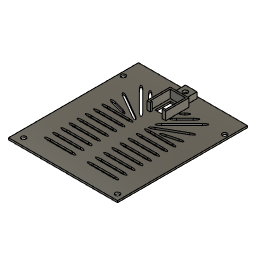
CaseBack (Autodesk Fusion 360 design; units mm, degrees)
Autodesk Fusion 360 part; units mm, degrees
(part 1 of 4)
sketch "Sketch1" plane through (0, 0, 0) normal (0, 0, 1) x (1, 0, 0)
  line L0 (0, 0) -> (94, 0)
  line L1 (94, 0) -> (94, 112.05)
  line L2 (94, 112.05) -> (0, 112.05)
  line L3 (0, 112.05) -> (0, 0)
  line L4 (0, 112.05) -> (3.5, 112.05)
  line L5 (3.5, 112.05) -> (3.5, 95.55)
  line L6 (3.5, 95.55) -> (0, 95.55)
  line L7 (0, 95.55) -> (0, 112.05)
  circle A0 centre (3.5, 95.55) radius 2
  line L8 (94, 112.05) -> (90.5, 112.05)
  line L9 (90.5, 112.05) -> (90.5, 95.55)
  line L10 (90.5, 95.55) -> (94, 95.55)
  line L11 (94, 95.55) -> (94, 112.05)
  circle A1 centre (90.5, 95.55) radius 2
  line L12 (0, 0) -> (5, 0)
  line L13 (5, 0) -> (5, 5)
  line L14 (5, 5) -> (0, 5)
  line L15 (0, 5) -> (0, 0)
  circle A2 centre (5, 5) radius 2
  line L16 (94, 0) -> (87.5, 0)
  line L17 (87.5, 0) -> (87.5, 6.5)
  line L18 (87.5, 6.5) -> (94, 6.5)
  line L19 (94, 6.5) -> (94, 0)
  circle A3 centre (87.5, 6.5) radius 2
  line L20 (0, 112.05) -> (0.25, 112.05)
  line L21 (0.25, 112.05) -> (0.25, 111.8)
  line L22 (0.25, 111.8) -> (0, 111.8)
  line L23 (0, 111.8) -> (0, 112.05)
  line L24 (94, 0) -> (93.75, 0)
  line L25 (93.75, 0) -> (93.75, 0.25)
  line L26 (93.75, 0.25) -> (94, 0.25)
  line L27 (94, 0.25) -> (94, 0)
  line L28 (93.75, 0.25) -> (0.25, 0.25)
  line L29 (0.25, 0.25) -> (0.25, 111.8)
  line L30 (0.25, 111.8) -> (93.75, 111.8)
  line L31 (93.75, 111.8) -> (93.75, 0.25)
  dimension "d1" = 94
  dimension "d2" = 112.05
  dimension "d3" = 3.5
  dimension "d4" = 16.5
  dimension "d5" = 4
  dimension "d6" = 3.5
  dimension "d7" = 16.5
  dimension "d8" = 4
  dimension "d9" = 5
  dimension "d10" = 5
  dimension "d11" = 4
  dimension "d12" = 6.5
  dimension "d13" = 6.5
  dimension "d14" = 4
  dimension "d15" = 0.25
  dimension "d16" = 0.25
  dimension "d17" = 0.25
  dimension "d18" = 0.25
  constraint horizontal L0
  constraint vertical L1
  constraint horizontal L2
  constraint vertical L3
  constraint horizontal L4
  constraint vertical L5
  constraint horizontal L6
  constraint vertical L7
  constraint coincident L5.end L6.start
  constraint horizontal L8
  constraint vertical L9
  constraint horizontal L10
  constraint vertical L11
  constraint coincident L9.end L10.start
  constraint horizontal L12
  constraint vertical L13
  constraint horizontal L14
  constraint vertical L15
  constraint coincident L13.end L14.start
  constraint horizontal L16
  constraint vertical L17
  constraint horizontal L18
  constraint vertical L19
  constraint coincident L17.end L18.start
  constraint horizontal L20
  constraint vertical L21
  constraint horizontal L22
  constraint vertical L23
  constraint horizontal L24
  constraint vertical L25
  constraint horizontal L26
  constraint vertical L27
  constraint horizontal L28
  constraint vertical L29
  constraint horizontal L30
  constraint vertical L31
  measures "d1" distance of L0.start L0.end
  measures "d2" distance of L0.start L2.end
  measures "d3" distance of L2.end L4.end
  measures "d4" distance of L2.end L6.end
  measures "d5" diameter of A0
  measures "d6" distance of L1.end L8.end
  measures "d7" distance of L1.end L10.end
  measures "d8" diameter of A1
  measures "d9" distance of L0.start L12.end
  measures "d10" distance of L0.start L14.end
  measures "d11" diameter of A2
  measures "d12" distance of L0.end L16.end
  measures "d13" distance of L0.end L18.end
  measures "d14" diameter of A3
  measures "d15" distance of L2.end L20.end
  measures "d16" distance of L2.end L22.end
  measures "d17" distance of L0.end L24.end
  measures "d18" distance of L0.end L26.end
extrude "Extrude1" add sketch "Sketch1" along normal blind 1.5 contours L13 L14 A2 L28 L29 | L5 L6 A0 L9 L10 A1 L13 L14 A2 L17 L18 A3 L28 L29 L30 L31 | L17 L18 A3 L28 L31 | L5 L6 A0 L29 L30 | L9 L10 A1 L30 L31
sketch "Sketch2" plane through (0, 0, 1.5) normal (0, 0, 1) x (-1, 0, 0)
  circle A0 centre (-87.5, -6.5) radius 2
  circle A1 centre (-90.5, -95.55) radius 2
  circle A2 centre (-3.5, -95.55) radius 2
  circle A3 centre (-5, -5) radius 2
  line L0 (-93.75, -111.8) -> (-0.25, -111.8)
  line L1 (-0.25, -111.8) -> (-0.25, -0.25)
  line L2 (-0.25, -0.25) -> (-93.75, -0.25)
  line L3 (-93.75, -0.25) -> (-93.75, -111.8)
  line L4 (-3.5, -95.55) -> (-8.5, -95.55)
  line L5 (-5, -5) -> (-10, -5)
  line L6 (-10, -5) -> (-10, -95.55)
  line L7 (-10, -95.55) -> (-8.5, -95.55)
  line L8 (-10, -111.8) -> (-10, -106.8)
  line L9 (-87.5, -6.5) -> (-82.5, -6.5)
  line L10 (-90.5, -95.55) -> (-85.5, -95.55)
  line L11 (-82.5, -6.5) -> (-82.5, -95.55)
  line L12 (-82.5, -95.55) -> (-85.5, -95.55)
  line L13 (-82.5, -111.8) -> (-82.5, -106.8)
  line L14 (-10, -106.8) -> (-82.5, -106.8)
  line L15 (-82.5, -106.8) -> (-82.5, -6.5)
  line L16 (-82.5, -6.5) -> (-10, -6.5)
  line L17 (-10, -6.5) -> (-10, -106.8)
  line L18 (-82.5, -6.5) -> (-82.5, -0.25)
  line L19 (-82.5, -0.25) -> (-82.5, -5.25)
  line L20 (-82.5, -5.25) -> (-10, -5.25)
  line L21 (-10, -5.25) -> (-10, -6.5)
  line L22 (-10, -6.5) -> (-82.5, -6.5)
  line L23 (-82.5, -6.5) -> (-82.5, -5.25)
  dimension "d21" = 5
  dimension "d22" = 5
  dimension "d23" = 5
  dimension "d24" = 5
  dimension "d25" = 5
  dimension "d26" = 5
  constraint coincident A2.centre L4.start
  constraint horizontal L4
  constraint coincident A3.centre L5.start
  constraint horizontal L5
  constraint perpendicular L4 L6
  constraint perpendicular L6 L7
  constraint coincident L0 L8.start
  constraint perpendicular L0 L8
  constraint coincident A0.centre L9.start
  constraint horizontal L9
  constraint coincident A1.centre L10.start
  constraint horizontal L10
  constraint perpendicular L10 L11
  constraint perpendicular L11 L12
  constraint coincident L0 L13.start
  constraint perpendicular L0 L13
  constraint horizontal L14
  constraint vertical L15
  constraint horizontal L16
  constraint vertical L17
  constraint coincident L2 L18.end
  constraint perpendicular L2 L18
  constraint perpendicular L2 L19
  constraint horizontal L20
  constraint vertical L21
  constraint horizontal L22
  constraint vertical L23
  measures "d21" distance of A2.centre L4.end
  measures "d22" distance of L8.start L8.end
  measures "d23" distance of A0.centre L9.end
  measures "d24" distance of A1.centre L10.end
  measures "d25" distance of L13.start L13.end
  measures "d26" distance of L18.end L19.end
extrude "Extrude2" cut sketch "Sketch2" against normal blind 12 contours L6 L11 L14 L15 L16 L17 L22 | L6 L16 L18 L20 L21 L22 L23
extrude "Extrude3" add 1 faces at (10, 39.1, 1) along direction (1, 0, 0) blind 72.5
sketch "Sketch3" plane through (0, 0, 1.5) normal (0, 0, 1) x (-1, 0, 0)
  circle A0 centre (-87.5, -6.5) radius 2
  circle A1 centre (-90.5, -95.55) radius 2
  circle A2 centre (-3.5, -95.55) radius 2
  circle A3 centre (-5, -5) radius 2
  line L0 (-93.75, -111.8) -> (-0.25, -111.8)
  line L1 (-0.25, -111.8) -> (-0.25, -0.25)
  line L2 (-0.25, -0.25) -> (-93.75, -0.25)
  line L3 (-93.75, -0.25) -> (-93.75, -111.8)
  line L4 (-0.25, -111.8) -> (-15.25, -111.8)
  line L5 (-15.25, -111.8) -> (-15.25, -0.25)
  line L6 (-15.25, -0.25) -> (-0.25, -0.25)
  line L7 (-0.25, -0.25) -> (-0.25, -111.8)
  line L8 (-93.75, -111.8) -> (-78.75, -111.8)
  line L9 (-78.75, -111.8) -> (-78.75, -0.25)
  line L10 (-78.75, -0.25) -> (-93.75, -0.25)
  line L11 (-93.75, -0.25) -> (-93.75, -111.8)
  line L12 (-78.75, -0.25) -> (-15.25, -0.25)
  line L13 (-15.25, -0.25) -> (-15.25, -15.25)
  line L14 (-15.25, -15.25) -> (-78.75, -15.25)
  line L15 (-78.75, -15.25) -> (-78.75, -0.25)
  line L16 (-15.25, -111.8) -> (-78.75, -111.8)
  line L17 (-78.75, -111.8) -> (-78.75, -96.8)
  line L18 (-78.75, -96.8) -> (-15.25, -96.8)
  line L19 (-15.25, -96.8) -> (-15.25, -111.8)
  line L20 (-47, -96.8) -> (-42.5, -96.8)
  line L21 (-42.5, -96.8) -> (-42.5, -83.8)
  line L22 (-42.5, -83.8) -> (-47, -83.8)
  line L23 (-47, -83.8) -> (-47, -96.8)
  line L24 (-47, -96.8) -> (-51.5, -96.8)
  line L25 (-51.5, -96.8) -> (-51.5, -83.8)
  line L26 (-51.5, -83.8) -> (-47, -83.8)
  line L27 (-47, -83.8) -> (-47, -96.8)
  dimension "d31" = 15
  dimension "d32" = 15
  dimension "d33" = 15
  dimension "d34" = 15
  dimension "d35" = 4.5
  dimension "d36" = 13
  dimension "d37" = 4.5
  dimension "d38" = 13
  constraint horizontal L4
  constraint vertical L5
  constraint horizontal L6
  constraint vertical L7
  constraint coincident L2 L5.end
  constraint coincident L0.end L1.start
  constraint horizontal L8
  constraint vertical L9
  constraint horizontal L10
  constraint vertical L11
  constraint coincident L0.start L3.end
  constraint horizontal L12
  constraint vertical L13
  constraint horizontal L14
  constraint vertical L15
  constraint horizontal L16
  constraint vertical L17
  constraint horizontal L18
  constraint vertical L19
  constraint horizontal L20
  constraint vertical L21
  constraint horizontal L22
  constraint vertical L23
  constraint midpoint L18 L20.start
  constraint horizontal L24
  constraint vertical L25
  constraint horizontal L26
  constraint vertical L27
  measures "d31" distance of L0.end L4.end
  measures "d32" distance of L0.start L8.end
  measures "d33" distance of L9.end L14.end
  measures "d34" distance of L4.end L18.end
  measures "d35" distance of L20.start L20.end
  measures "d36" distance of L20.start L22.end
  measures "d37" distance of L20.start L24.end
  measures "d38" distance of L20.start L22.end
extrude "Extrude4" cut sketch "Sketch3" against normal blind 40 contours L18 L23 L24 L25 L26 L27 | L18 L20 L21 L22 L23 L27
sketch "Sketch4" plane through (0, 0, 1.5) normal (0, 0, 1) x (-1, 0, 0)
  line L0 (-42.5, -83.8) -> (-42.5, -96.8)
  line L1 (-42.5, -96.8) -> (-51.5, -96.8)
  line L2 (-51.5, -96.8) -> (-51.5, -83.8)
  line L3 (-51.5, -83.8) -> (-42.5, -83.8)
  circle A0 centre (-87.5, -6.5) radius 2
  circle A1 centre (-90.5, -95.55) radius 2
  circle A2 centre (-3.5, -95.55) radius 2
  circle A3 centre (-5, -5) radius 2
  line L4 (-93.75, -111.8) -> (-0.25, -111.8)
  line L5 (-0.25, -111.8) -> (-0.25, -0.25)
  line L6 (-0.25, -0.25) -> (-93.75, -0.25)
  line L7 (-93.75, -0.25) -> (-93.75, -111.8)
  line L8 (-42.5, -96.8) -> (-40.5, -96.8)
  line L9 (-40.5, -96.8) -> (-40.5, -98.8)
  line L10 (-40.5, -98.8) -> (-42.5, -98.8)
  line L11 (-42.5, -98.8) -> (-42.5, -96.8)
  line L12 (-51.5, -83.8) -> (-53.5, -83.8)
  line L13 (-53.5, -83.8) -> (-53.5, -81.8)
  line L14 (-53.5, -81.8) -> (-51.5, -81.8)
  line L15 (-51.5, -81.8) -> (-51.5, -83.8)
  line L16 (-40.5, -98.8) -> (-53.5, -98.8)
  line L17 (-53.5, -98.8) -> (-53.5, -81.8)
  line L18 (-53.5, -81.8) -> (-40.5, -81.8)
  line L19 (-40.5, -81.8) -> (-40.5, -98.8)
  line L20 (-40.5, -98.8) -> (-39, -98.8)
  line L21 (-39, -98.8) -> (-39, -100.3)
  line L22 (-39, -100.3) -> (-40.5, -100.3)
  line L23 (-40.5, -100.3) -> (-40.5, -98.8)
  line L24 (-53.5, -81.8) -> (-55, -81.8)
  line L25 (-55, -81.8) -> (-55, -80.3)
  line L26 (-55, -80.3) -> (-53.5, -80.3)
  line L27 (-53.5, -80.3) -> (-53.5, -81.8)
  line L28 (-55, -80.3) -> (-39, -80.3)
  line L29 (-39, -80.3) -> (-39, -100.3)
  line L30 (-39, -100.3) -> (-55, -100.3)
  line L31 (-55, -100.3) -> (-55, -80.3)
  line L32 (-40.5, -81.8) -> (-42, -81.8)
  line L33 (-42, -81.8) -> (-42, -80.3)
  line L34 (-42, -80.3) -> (-40.5, -80.3)
  line L35 (-40.5, -80.3) -> (-40.5, -81.8)
  line L36 (-53.5, -81.8) -> (-52, -81.8)
  line L37 (-52, -81.8) -> (-52, -80.3)
  line L38 (-52, -80.3) -> (-53.5, -80.3)
  line L39 (-53.5, -80.3) -> (-53.5, -81.8)
  dimension "d41" = 2
  dimension "d42" = 2
  dimension "d43" = 2
  dimension "d44" = 2
  dimension "d45" = 1.5
  dimension "d46" = 1.5
  dimension "d47" = 1.5
  dimension "d48" = 1.5
  dimension "d49" = 1.5
  dimension "d50" = 1.5
  constraint horizontal L8
  constraint vertical L9
  constraint horizontal L10
  constraint vertical L11
  constraint coincident L0.end L1.start
  constraint horizontal L12
  constraint vertical L13
  constraint horizontal L14
  constraint vertical L15
  constraint coincident L2.end L3.start
  constraint horizontal L16
  constraint vertical L17
  constraint horizontal L18
  constraint vertical L19
  constraint horizontal L20
  constraint vertical L21
  constraint horizontal L22
  constraint vertical L23
  constraint horizontal L24
  constraint vertical L25
  constraint horizontal L26
  constraint vertical L27
  constraint horizontal L28
  constraint vertical L29
  constraint horizontal L30
  constraint vertical L31
  constraint horizontal L32
  constraint vertical L33
  constraint horizontal L34
  constraint vertical L35
  constraint horizontal L36
  constraint vertical L37
  constraint horizontal L38
  constraint vertical L39
  measures "d41" distance of L0.end L8.end
  measures "d42" distance of L0.end L10.end
  measures "d43" distance of L2.end L12.end
  measures "d44" distance of L2.end L14.end
  measures "d45" distance of L9.end L20.end
  measures "d46" distance of L9.end L22.end
  measures "d47" distance of L13.end L24.end
  measures "d48" distance of L13.end L26.end
  measures "d49" distance of L18.end L32.end
  measures "d50" distance of L13.end L36.end
extrude "Extrude5" add sketch "Sketch4" along normal blind 7 contours L9 L19 L20 L28 L29 L35 | L10 L13 L16 L17 L23 L24 L30 L31 | L20 L21 L22 L23 L29 L30 | L18 L28 L32 L33 L34 L35 | L14 L18 L27 L28 L36 L37 L38 L39 | L24 L25 L26 L27 L28 L31 L39
sketch "Sketch5" plane through (0, 0, 1.5) normal (0, 0, 1) x (-1, 0, 0)
  line L0 (-40.5, -81.8) -> (-42, -81.8)
  line L1 (-42, -81.8) -> (-42, -80.3)
  line L2 (-42, -80.3) -> (-39, -80.3)
  line L3 (-39, -80.3) -> (-39, -100.3)
  line L4 (-39, -100.3) -> (-55, -100.3)
  line L5 (-55, -100.3) -> (-55, -80.3)
  line L6 (-55, -80.3) -> (-52, -80.3)
  line L7 (-52, -80.3) -> (-52, -81.8)
  line L8 (-52, -81.8) -> (-53.5, -81.8)
  line L9 (-53.5, -81.8) -> (-53.5, -98.8)
  line L10 (-53.5, -98.8) -> (-40.5, -98.8)
  line L11 (-40.5, -98.8) -> (-40.5, -81.8)
  line L12 (-42.5, -83.8) -> (-42.5, -96.8)
  line L13 (-42.5, -96.8) -> (-51.5, -96.8)
  line L14 (-51.5, -96.8) -> (-51.5, -83.8)
  line L15 (-51.5, -83.8) -> (-42.5, -83.8)
  circle A0 centre (-87.5, -6.5) radius 2
  circle A1 centre (-90.5, -95.55) radius 2
  circle A2 centre (-3.5, -95.55) radius 2
  circle A3 centre (-5, -5) radius 2
  line L16 (-93.75, -111.8) -> (-0.25, -111.8)
  line L17 (-0.25, -111.8) -> (-0.25, -0.25)
  line L18 (-0.25, -0.25) -> (-93.75, -0.25)
  line L19 (-93.75, -0.25) -> (-93.75, -111.8)
  line L20 (-47, -100.3) -> (-42, -100.3)
  line L21 (-42, -100.3) -> (-42, -110.3)
  line L22 (-42, -110.3) -> (-47, -110.3)
  line L23 (-47, -110.3) -> (-47, -100.3)
  line L24 (-42, -110.3) -> (-52, -110.3)
  line L25 (-52, -110.3) -> (-52, -100.3)
  line L26 (-52, -100.3) -> (-42, -100.3)
  line L27 (-42, -100.3) -> (-42, -110.3)
  line L28 (-42, -110.3) -> (-52, -100.3)
  circle A4 centre (-47, -105.3) radius 2
  line L29 (-43.9689, -107.05) -> (-43.9689, -103.55)
  line L30 (-43.9689, -103.55) -> (-47, -101.8)
  line L31 (-47, -101.8) -> (-50.0311, -103.55)
  line L32 (-50.0311, -103.55) -> (-50.0311, -107.05)
  line L33 (-50.0311, -107.05) -> (-47, -108.8)
  line L34 (-47, -108.8) -> (-43.9689, -107.05)
  line L35 (-43.9689, -107.05) -> (-43.9689, -110.3)
  line L36 (-50.0311, -107.05) -> (-50.0311, -110.3)
  point P0 (-47, -105.3)
  dimension "d53" = 5
  dimension "d54" = 10
  dimension "d55" = 10
  dimension "d56" = 10
  dimension "d57" = 4
  dimension "d58" = 3.5
  constraint horizontal L20
  constraint vertical L21
  constraint horizontal L22
  constraint vertical L23
  constraint midpoint L4 L20.start
  constraint horizontal L24
  constraint vertical L25
  constraint horizontal L26
  constraint vertical L27
  constraint midpoint L28 P0
  constraint vertical L35
  constraint coincident L22 L35.end
  constraint coincident L24 L36.end
  constraint perpendicular L24 L36
  measures "d53" distance of L20.start L20.end
  measures "d54" distance of L20.start L22.end
  measures "d55" distance of L21.end L24.end
  measures "d56" distance of L21.end L20.end
  measures "d57" diameter of A4
  measures "d58" distance of L29.start L29.end
extrude "Extrude6" add sketch "Sketch5" along normal blind 2 contours L4 L20 L21 L23 L26 L27 L28 L29 L30 L35 | L4 L23 L26 L28 L31 | L22 L24 L28 L35 | L24 L25 L28 L31 L32 L36 | L23 L28 A4 | L23 L28 A4 | L23 L28 A4 | L23 L28 A4
extrude "Extrude7" add 1 faces at (44.323, 101.8833, 3.5) along direction (0, 0, 1) blind 1
sketch "Sketch6" plane through (0, 100.3, 0) normal (0, 1, 0) x (-1, 0, 0)
  line L0 (-52, 1.5) -> (-52, 4.5)
  line L1 (-52, 4.5) -> (-42, 4.5)
  line L2 (-42, 4.5) -> (-42, 1.5)
  line L3 (-42, 1.5) -> (-39, 1.5)
  line L4 (-39, 1.5) -> (-39, 8.5)
  line L5 (-39, 8.5) -> (-55, 8.5)
  line L6 (-55, 8.5) -> (-55, 1.5)
  line L7 (-55, 1.5) -> (-52, 1.5)
  line L8 (-52, 4.5) -> (-42, 4.5)
  line L9 (-42, 4.5) -> (-42, 6.5)
  line L10 (-42, 6.5) -> (-52, 6.5)
  line L11 (-52, 6.5) -> (-52, 4.5)
  dimension "d63" = 2
  constraint horizontal L8
  constraint vertical L9
  constraint horizontal L10
  constraint vertical L11
  constraint coincident L0.end L1.start
  measures "d63" distance of L0.end L10.end
extrude "Extrude8" add sketch "Sketch6" along normal blind 10 contours L1 L8 L9 L10 L11
extrude "Extrude9" cut 1 faces at (47.6006, 105.0107, 3.5) along direction (0, 0, 1) blind 6
extrude "Extrude10" cut 1 faces at (47.6006, 105.0107, 3.5) along direction (0, 0, -1) blind 2
sketch "Sketch7" plane through (0, 0, 1.5) normal (0, 0, 1) x (-1, 0, 0)
  line L0 (-93.75, -111.8) -> (-0.25, -111.8)
  line L1 (-0.25, -111.8) -> (-0.25, -0.25)
  line L2 (-0.25, -0.25) -> (-93.75, -0.25)
  line L3 (-93.75, -0.25) -> (-93.75, -111.8)
  circle A0 centre (-5, -5) radius 2
  circle A1 centre (-3.5, -95.55) radius 2
  circle A2 centre (-90.5, -95.55) radius 2
  circle A3 centre (-87.5, -6.5) radius 2
  line L4 (-42.5, -83.8) -> (-42.5, -96.8)
  line L5 (-42.5, -96.8) -> (-51.5, -96.8)
  line L6 (-51.5, -96.8) -> (-51.5, -83.8)
  line L7 (-51.5, -83.8) -> (-42.5, -83.8)
  line L8 (-42, -100.3) -> (-42, -110.3)
  line L9 (-42, -110.3) -> (-43.9689, -110.3)
  line L10 (-43.9689, -110.3) -> (-43.9689, -103.55)
  line L11 (-43.9689, -103.55) -> (-47, -101.8)
  line L12 (-47, -101.8) -> (-50.0311, -103.55)
  line L13 (-50.0311, -103.55) -> (-50.0311, -110.3)
  line L14 (-50.0311, -110.3) -> (-52, -110.3)
  line L15 (-52, -110.3) -> (-52, -100.3)
  line L16 (-52, -100.3) -> (-55, -100.3)
  line L17 (-55, -100.3) -> (-55, -80.3)
  line L18 (-55, -80.3) -> (-52, -80.3)
  line L19 (-52, -80.3) -> (-52, -81.8)
  line L20 (-52, -81.8) -> (-53.5, -81.8)
  line L21 (-53.5, -81.8) -> (-53.5, -98.8)
  line L22 (-53.5, -98.8) -> (-40.5, -98.8)
  line L23 (-40.5, -98.8) -> (-40.5, -81.8)
  line L24 (-40.5, -81.8) -> (-42, -81.8)
  line L25 (-42, -81.8) -> (-42, -80.3)
  line L26 (-42, -80.3) -> (-39, -80.3)
  line L27 (-39, -80.3) -> (-39, -100.3)
  line L28 (-39, -100.3) -> (-42, -100.3)
  line L29 (-0.25, -111.8) -> (-15.25, -111.8)
  line L30 (-15.25, -111.8) -> (-15.25, -96.8)
  line L31 (-15.25, -96.8) -> (-0.25, -96.8)
  line L32 (-0.25, -96.8) -> (-0.25, -111.8)
  line L33 (-93.75, -111.8) -> (-78.75, -111.8)
  line L34 (-78.75, -111.8) -> (-78.75, -96.8)
  line L35 (-78.75, -96.8) -> (-93.75, -96.8)
  line L36 (-93.75, -96.8) -> (-93.75, -111.8)
  line L37 (-0.25, -0.25) -> (-15.25, -0.25)
  line L38 (-15.25, -0.25) -> (-15.25, -15.25)
  line L39 (-15.25, -15.25) -> (-0.25, -15.25)
  line L40 (-0.25, -15.25) -> (-0.25, -0.25)
  line L41 (-93.75, -0.25) -> (-78.75, -0.25)
  line L42 (-78.75, -0.25) -> (-78.75, -15.25)
  line L43 (-78.75, -15.25) -> (-93.75, -15.25)
  line L44 (-93.75, -15.25) -> (-93.75, -0.25)
  line L45 (-15.25, -96.8) -> (-78.75, -96.8)
  line L46 (-78.75, -96.8) -> (-78.75, -15.25)
  line L47 (-78.75, -15.25) -> (-15.25, -15.25)
  line L48 (-15.25, -15.25) -> (-15.25, -96.8)
  line L49 (-47, -96.8) -> (-42, -96.8)
  line L50 (-42, -96.8) -> (-42, -15.25)
  line L51 (-42, -15.25) -> (-47, -15.25)
  line L52 (-47, -15.25) -> (-47, -96.8)
  line L53 (-47, -96.8) -> (-52.5668, -96.8)
  line L54 (-52.5668, -96.8) -> (-52.5668, -15.25)
  line L55 (-52.5668, -15.25) -> (-47, -15.25)
  line L56 (-47, -15.25) -> (-47, -96.8)
  line L57 (-39, -96.8) -> (-34, -96.8)
  line L58 (-34, -96.8) -> (-39.1645, -91.6355)
  line L59 (-34, -96.8) -> (-26.6963, -96.8) construction
  line L60 (-34, -96.8) -> (-32.5858, -95.3858)
  line L61 (-39.1645, -91.6355) -> (-37.7503, -90.2213)
  line L62 (-32.5858, -95.3858) -> (-37.7503, -90.2213)
  line L63 (-32.5858, -95.3858) -> (-31.1716, -96.8)
  line L64 (-32.5858, -95.3858) -> (-30.5858, -95.3858) construction
  line L65 (-31.1716, -96.8) -> (-26.1716, -96.8)
  line L66 (-26.6963, -96.8) -> (-39, -84.4963)
  line L67 (-26.6963, -96.8) -> (-9.2963, -96.8) construction
  line L68 (-26.6963, -96.8) -> (-25.2821, -95.3858)
  line L69 (-39, -84.4963) -> (-37.5858, -83.0821)
  line L70 (-37.5858, -83.0821) -> (-25.2821, -95.3858)
  line L71 (-25.2821, -95.3858) -> (-23.8679, -96.8)
  line L72 (-25.2821, -95.3858) -> (-23.2821, -95.3858) construction
  line L73 (-23.8679, -96.8) -> (-18.8679, -96.8)
  line L74 (-18.8679, -96.8) -> (-42, -73.6679)
  line L75 (-18.8679, -96.8) -> (13.8458, -96.8) construction
  line L76 (-18.8679, -96.8) -> (-17.4537, -95.3858)
  line L77 (-17.4537, -95.3858) -> (-42, -70.8395)
  line L78 (-42, -73.6679) -> (-40.5858, -72.2537)
  line L79 (-39, -84.4963) -> (-42, -81.4963)
  line L80 (-39, -84.4963) -> (-34.7574, -84.4963) construction
  line L81 (-39.1645, -91.6355) -> (-42, -88.8)
  line L82 (-17.4537, -95.3858) -> (-16.0395, -96.8)
  line L83 (-17.4537, -95.3858) -> (-15.4537, -95.3858) construction
  line L84 (-17.4537, -95.3858) -> (-15.4537, -95.3858) construction
  line L85 (-25.2821, -95.3858) -> (-23.2821, -95.3858) construction
  line L86 (-47, -96.8) -> (-42, -96.8)
  line L87 (-32.5858, -95.3858) -> (-30.5858, -95.3858) construction
  line L88 (-18.8679, -96.8) -> (-42, -73.6679)
  line L89 (-32.5858, -95.3858) -> (-31.1716, -96.8)
  line L90 (-39, -84.4963) -> (-34.7574, -84.4963) construction
  line L91 (-26.6963, -96.8) -> (-39, -84.4963)
  line L92 (-34, -96.8) -> (-32.5858, -95.3858)
  line L93 (-42, -73.6679) -> (-40.5858, -72.2537)
  line L94 (-17.4537, -95.3858) -> (-42, -70.8395)
  line L95 (-25.2821, -95.3858) -> (-23.8679, -96.8)
  line L96 (-32.5858, -95.3858) -> (-37.7503, -90.2213)
  line L97 (-18.8679, -96.8) -> (-17.4537, -95.3858)
  line L98 (-37.5858, -83.0821) -> (-25.2821, -95.3858)
  line L99 (-39, -84.4963) -> (-42, -81.4963)
  line L100 (-31.1716, -96.8) -> (-26.1716, -96.8)
  line L101 (-26.6963, -96.8) -> (-25.2821, -95.3858)
  line L102 (-26.6963, -96.8) -> (-9.2963, -96.8) construction
  line L103 (-17.4537, -95.3858) -> (-16.0395, -96.8)
  line L104 (-39.1645, -91.6355) -> (-42, -88.8)
  line L105 (-34, -96.8) -> (-26.6963, -96.8) construction
  line L106 (-39, -84.4963) -> (-37.5858, -83.0821)
  line L107 (-34, -96.8) -> (-39.1645, -91.6355)
  line L108 (-23.8679, -96.8) -> (-18.8679, -96.8)
  line L109 (-39, -96.8) -> (-34, -96.8)
  line L110 (-39.1645, -91.6355) -> (-37.7503, -90.2213)
  line L111 (-55, -96.8) -> (-60, -96.8)
  line L112 (-60, -96.8) -> (-55, -91.8)
  line L113 (-60, -96.8) -> (-52.9289, -96.8) construction
  line L114 (-55, -91.8) -> (-56.4142, -90.3858)
  line L115 (-56.4142, -90.3858) -> (-62.8284, -96.8)
  line L116 (-60, -96.8) -> (-61.4142, -95.3858)
  line L117 (-62.8284, -96.8) -> (-67.8284, -96.8)
  line L118 (-67.8284, -96.8) -> (-55, -83.9716)
  line L119 (-67.8284, -96.8) -> (-49.6863, -96.8) construction
  line L120 (-55, -83.9716) -> (-56.4142, -82.5574)
  line L121 (-56.4142, -82.5574) -> (-70.6569, -96.8)
  line L122 (-67.8284, -96.8) -> (-69.2426, -95.3858)
  line L123 (-70.6569, -96.8) -> (-75.6569, -96.8)
  line L124 (-75.6569, -96.8) -> (-52.5668, -73.71)
  line L125 (-75.6569, -96.8) -> (-43.0026, -96.8) construction
  line L126 (-52.5668, -73.71) -> (-53.981, -72.2958)
  line L127 (-53.981, -72.2958) -> (-78.4853, -96.8)
  line L128 (-53.981, -72.2958) -> (-19.3268, -72.2958) construction
  line L129 (-75.6569, -96.8) -> (-77.0711, -95.3858)
  line L130 (-18.8679, -96.8) -> (-21.6963, -93.9716)
  line L131 (-21.6963, -93.9716) -> (-20.2821, -92.5574)
  ellipse E0 centre (-20.9892, -93.2645) end of major axis (-21.6963, -93.9716) minor radius 4
  line L132 (-20.2821, -92.5574) -> (-21.6963, -93.9716)
  line L133 (-23.8177, -90.436) -> (-18.1608, -96.0929)
  line L134 (-42, -73.6679) -> (-39.1716, -76.4963)
  line L135 (-39.1716, -76.4963) -> (-37.7574, -75.0821)
  line L136 (-39, -84.4963) -> (-36.1716, -87.3248)
  line L137 (-36.1716, -87.3248) -> (-34.7574, -85.9106)
  line L138 (-26.6963, -96.8) -> (-29.5248, -93.9716)
  line L139 (-29.5248, -93.9716) -> (-28.1106, -92.5574)
  line L140 (-34, -96.8) -> (-36.8284, -93.9716)
  line L141 (-36.8284, -93.9716) -> (-35.4142, -92.5574)
  line L142 (-39.1645, -91.6355) -> (-36.336, -94.464)
  line L143 (-36.336, -94.464) -> (-34.9218, -93.0497)
  ellipse E1 centre (-38.4645, -75.7892) end of major axis (-39.1716, -76.4963) minor radius 4
  line L144 (-37.7574, -75.0821) -> (-39.1716, -76.4963)
  line L145 (-41.2929, -72.9608) -> (-35.636, -78.6177)
  ellipse E2 centre (-28.8177, -93.2645) end of major axis (-29.5248, -93.9716) minor radius 4
  line L146 (-28.1106, -92.5574) -> (-29.5248, -93.9716)
  line L147 (-31.6461, -90.436) -> (-25.9892, -96.0929)
  ellipse E3 centre (-35.4645, -86.6177) end of major axis (-36.1716, -87.3248) minor radius 4
  line L148 (-34.7574, -85.9106) -> (-36.1716, -87.3248)
  line L149 (-38.2929, -83.7892) -> (-32.636, -89.4461)
  ellipse E4 centre (-35.6289, -93.7569) end of major axis (-36.336, -94.464) minor radius 4
  line L150 (-34.9218, -93.0497) -> (-36.336, -94.464)
  line L151 (-38.4574, -90.9284) -> (-32.8005, -96.5853)
  ellipse E5 centre (-36.1213, -93.2645) end of major axis (-36.8284, -93.9716) minor radius 4
  line L152 (-35.4142, -92.5574) -> (-36.8284, -93.9716)
  line L153 (-38.9497, -90.436) -> (-33.2929, -96.0929)
  line L154 (-52.5668, -73.71) -> (-55.3953, -76.5384)
  line L155 (-55.3953, -76.5384) -> (-56.8095, -75.1242)
  line L156 (-55, -83.9716) -> (-57.8284, -86.8)
  line L157 (-57.8284, -86.8) -> (-59.2426, -85.3858)
  line L158 (-55, -91.8) -> (-57.8284, -94.6284)
  line L159 (-57.8284, -94.6284) -> (-59.2426, -93.2142)
  line L160 (-60, -96.8) -> (-57.1716, -93.9716)
  line L161 (-57.1716, -93.9716) -> (-58.5858, -92.5574)
  line L162 (-67.8284, -96.8) -> (-65, -93.9716)
  line L163 (-65, -93.9716) -> (-66.4142, -92.5574)
  line L164 (-75.6569, -96.8) -> (-72.8284, -93.9716)
  line L165 (-72.8284, -93.9716) -> (-74.2426, -92.5574)
  ellipse E6 centre (-56.1024, -75.8313) end of major axis (-55.3953, -76.5384) minor radius 4
  line L166 (-56.8095, -75.1242) -> (-55.3953, -76.5384)
  line L167 (-58.9308, -78.6597) -> (-53.2739, -73.0029)
  ellipse E7 centre (-58.5355, -86.0929) end of major axis (-57.8284, -86.8) minor radius 4
  line L168 (-59.2426, -85.3858) -> (-57.8284, -86.8)
  line L169 (-61.364, -88.9213) -> (-55.7071, -83.2645)
  ellipse E8 centre (-58.5355, -93.9213) end of major axis (-57.8284, -94.6284) minor radius 4
  line L170 (-59.2426, -93.2142) -> (-57.8284, -94.6284)
  line L171 (-61.364, -96.7497) -> (-55.7071, -91.0929)
  ellipse E9 centre (-57.8787, -93.2645) end of major axis (-57.1716, -93.9716) minor radius 4
  line L172 (-58.5858, -92.5574) -> (-57.1716, -93.9716)
  line L173 (-60.7071, -96.0929) -> (-55.0503, -90.436)
  ellipse E10 centre (-65.7071, -93.2645) end of major axis (-65, -93.9716) minor radius 4
  line L174 (-66.4142, -92.5574) -> (-65, -93.9716)
  line L175 (-68.5355, -96.0929) -> (-62.8787, -90.436)
  ellipse E11 centre (-73.5355, -93.2645) end of major axis (-72.8284, -93.9716) minor radius 4
  line L176 (-74.2426, -92.5574) -> (-72.8284, -93.9716)
  line L177 (-76.364, -96.0929) -> (-70.7071, -90.436)
  point P0 (-15.25, -96.8)
  dimension "d70" = 15
  dimension "d71" = 15
  dimension "d72" = 15
  dimension "d73" = 15
  dimension "d74" = 15
  dimension "d75" = 15
  dimension "d76" = 15
  dimension "d77" = 15
  dimension "d78" = 5.5668
  dimension "d79" = 5
  dimension "d80" = 135
  dimension "d81" = 2
  dimension "d82" = 2
  dimension "d83" = 45
  dimension "d84" = 5
  dimension "d85" = 135
  dimension "d86" = 2
  dimension "d87" = 2
  dimension "d88" = 45
  dimension "d89" = 5
  dimension "d90" = 135
  dimension "d91" = 2
  dimension "d92" = 135
  dimension "d93" = 45
  dimension "d94" = 5
  dimension "d95" = 135
  dimension "d96" = 2
  dimension "d97" = 2
  dimension "d98" = 45
  dimension "d99" = 5
  dimension "d100" = 135
  dimension "d101" = 2
  dimension "d102" = 2
  dimension "d103" = 45
  dimension "d104" = 5
  dimension "d105" = 2
  dimension "d106" = 135
  dimension "d107" = 45
  dimension "d108" = 5
  dimension "d109" = 45
  dimension "d110" = 90
  dimension "d111" = 2
  dimension "d112" = 5
  dimension "d113" = 45
  dimension "d114" = 2
  dimension "d115" = 5
  dimension "d116" = 45
  dimension "d117" = 2
  dimension "d118" = 135
  dimension "d119" = 4
  dimension "d120" = 4
  dimension "d121" = 4
  dimension "d122" = 4
  dimension "d123" = 4
  dimension "d124" = 4
  dimension "d125" = 4
  dimension "d126" = 4
  dimension "d127" = 4
  dimension "d128" = 4
  dimension "d129" = 4
  dimension "d130" = 4
  constraint horizontal L29
  constraint vertical L30
  constraint horizontal L31
  constraint vertical L32
  constraint coincident L0.end L1.start
  constraint horizontal L33
  constraint vertical L34
  constraint horizontal L35
  constraint vertical L36
  constraint coincident L0.start L3.end
  constraint horizontal L37
  constraint vertical L38
  constraint horizontal L39
  constraint vertical L40
  constraint coincident L1.end L2.start
  constraint horizontal L41
  constraint vertical L42
  constraint horizontal L43
  constraint vertical L44
  constraint coincident L2.end L3.start
  constraint horizontal L45
  constraint vertical L46
  constraint horizontal L47
  constraint vertical L48
  constraint horizontal L49
  constraint vertical L50
  constraint horizontal L51
  constraint vertical L52
  constraint coincident L47 L50.end
  constraint midpoint L45 L49.start
  constraint horizontal L53
  constraint vertical L54
  constraint horizontal L55
  constraint vertical L56
  constraint coincident L47 L54.end
  constraint coincident L45 L57.start
  constraint coincident L27 L57.start
  constraint perpendicular L27 L57
  constraint horizontal L59
  constraint perpendicular L58 L60
  constraint perpendicular L58 L61
  constraint horizontal L64
  constraint coincident L45 L63.end
  constraint parallel L59 L65
  constraint horizontal L67
  constraint coincident L27 L66.end
  constraint perpendicular L66 L68
  constraint perpendicular L66 L69
  constraint horizontal L72
  constraint coincident L67 L71.end
  constraint parallel L45 L73
  constraint horizontal L75
  constraint coincident L50 L74.end
  constraint perpendicular L74 L76
  constraint coincident L50 L77.end
  constraint perpendicular L76 L77
  constraint coincident L77 L78.end
  constraint perpendicular L77 L78
  constraint horizontal L80
  constraint coincident L25 L79.end
  constraint coincident L50 L79.end
  constraint coincident L50 L81.end
  constraint perpendicular L61 L81
  constraint horizontal L83
  constraint coincident L67 L82.end
  constraint horizontal L86
  constraint horizontal L105
  constraint perpendicular L92 L107
  constraint perpendicular L107 L110
  constraint horizontal L87
  constraint parallel L100 L105
  constraint horizontal L102
  constraint perpendicular L91 L101
  constraint perpendicular L91 L106
  constraint horizontal L85
  constraint coincident L71.end L102
  constraint perpendicular L88 L97
  constraint perpendicular L94 L97
  constraint coincident L78.end L94
  constraint perpendicular L93 L94
  constraint horizontal L90
  constraint perpendicular L104 L110
  constraint horizontal L84
  constraint coincident L82.end L102
  constraint coincident L17 L111.start
  constraint coincident L45 L111.start
  constraint perpendicular L17 L111
  constraint horizontal L113
  constraint coincident L17 L112.end
  constraint coincident L45 L115.end
  constraint perpendicular L114 L115
  constraint coincident L115 L116.end
  constraint perpendicular L115 L116
  constraint parallel L45 L117
  constraint horizontal L119
  constraint coincident L17 L118.end
  constraint perpendicular L118 L120
  constraint coincident L45 L121.end
  constraint perpendicular L120 L121
  constraint coincident L121 L122.end
  constraint perpendicular L121 L122
  constraint parallel L45 L123
  constraint horizontal L125
  constraint coincident L54 L124.end
  constraint perpendicular L124 L126
  constraint horizontal L128
  constraint coincident L45 L127.end
  constraint coincident L127 L129.end
  constraint perpendicular L127 L129
  constraint coincident L88 L130.end
  constraint perpendicular L97 L130
  constraint coincident L94 L131.end
  constraint perpendicular L94 L131
  constraint midpoint L131 E0.centre
  constraint coincident L131.end E0
  constraint coincident L130.end E0
  constraint perpendicular L93 L134
  constraint coincident L77 L135.end
  constraint perpendicular L77 L135
  constraint perpendicular L135 L136
  constraint coincident L70 L137.end
  constraint perpendicular L70 L137
  constraint perpendicular L137 L138
  constraint coincident L70 L139.end
  constraint perpendicular L70 L139
  constraint perpendicular L92 L140
  constraint coincident L62 L141.end
  constraint perpendicular L62 L141
  constraint perpendicular L141 L142
  constraint coincident L96 L143.end
  constraint perpendicular L96 L143
  constraint midpoint L135 E1.centre
  constraint perpendicular L134 L144
  constraint coincident L135.end E1
  constraint coincident L134.end E1
  constraint midpoint L139 E2.centre
  constraint coincident L139.end E2
  constraint coincident L138.end E2
  constraint midpoint L137 E3.centre
  constraint coincident L137.end E3
  constraint coincident L136.end E3
  constraint midpoint L143 E4.centre
  constraint coincident L143.end E4
  constraint coincident L142.end E4
  constraint midpoint L141 E5.centre
  constraint coincident L141.end E5
  constraint coincident L140.end E5
  constraint perpendicular L126 L154
  constraint coincident L127 L155.end
  constraint perpendicular L127 L155
  constraint perpendicular L120 L156
  constraint coincident L121 L157.end
  constraint perpendicular L121 L157
  constraint perpendicular L114 L158
  constraint coincident L115 L159.end
  constraint perpendicular L115 L159
  constraint perpendicular L159 L160
  constraint coincident L115 L161.end
  constraint perpendicular L115 L161
  constraint perpendicular L161 L162
  constraint coincident L121 L163.end
  constraint perpendicular L121 L163
  constraint perpendicular L129 L164
  constraint coincident L127 L165.end
  constraint perpendicular L127 L165
  constraint midpoint L155 E6.centre
  constraint coincident L155.end E6
  constraint coincident L154.end E6
  constraint midpoint L157 E7.centre
  constraint coincident L157.end E7
  constraint coincident L156.end E7
  constraint midpoint L159 E8.centre
  constraint coincident L159.end E8
  constraint coincident L158.end E8
  constraint midpoint L161 E9.centre
  constraint coincident L161.end E9
  constraint coincident L160.end E9
  constraint midpoint L163 E10.centre
  constraint coincident L163.end E10
  constraint coincident L162.end E10
  constraint midpoint L165 E11.centre
  constraint coincident L165.end E11
  constraint coincident L164.end E11
  measures "d70" distance of L0.end L29.end
  measures "d71" distance of L0.end L31.end
  measures "d72" distance of L0.start L33.end
  measures "d73" distance of L0.start L35.end
  measures "d74" distance of L1.end L37.end
  measures "d75" distance of L1.end L39.end
  measures "d76" distance of L2.end L41.end
  measures "d77" distance of L2.end L43.end
  measures "d78" distance of L49.start L53.end
  measures "d79" distance of L57.start L57.end
  measures "d80" angle of L58 L59
  measures "d81" distance of L57.end L60.end
  measures "d82" distance of L58.end L61.end
  measures "d83" angle of L63 L64
  measures "d84" distance of L63.end L65.end
  measures "d85" angle of L66 L67
  measures "d86" distance of L59.end L68.end
  measures "d87" distance of L66.end L69.end
  measures "d88" angle of L71 L72
  measures "d89" distance of L71.end L73.end
  measures "d90" angle of L74 L75
  measures "d91" distance of L73.end L76.end
  measures "d92" angle of L79 L80
  measures "d93" angle of L82 L83
  measures "d94" distance of L57.start L57.end
  measures "d95" angle of L105 L107
  measures "d96" distance of L57.end L60.end
  measures "d97" distance of L58.end L61.end
  measures "d98" angle of L87 L89
  measures "d99" distance of L63.end L65.end
  measures "d100" angle of L91 L102
  measures "d101" distance of L68.end L59.end
  measures "d102" distance of L66.end L69.end
  measures "d103" angle of L85 L95
  measures "d104" distance of L73.end L71.end
  measures "d105" distance of L73.end L76.end
  measures "d106" angle of L90 L99
  measures "d107" angle of L84 L103
  measures "d108" distance of L111.start L111.end
  measures "d109" angle of L112 L113
  measures "d110" angle of L112 L114
  measures "d111" distance of L112.end L114.end
  measures "d112" distance of L115.end L117.end
  measures "d113" angle of L118 L119
  measures "d114" distance of L118.end L120.end
  measures "d115" distance of L121.end L123.end
  measures "d116" angle of L124 L125
  measures "d117" distance of L124.end L126.end
  measures "d118" angle of L127 L128
  measures "d119" distance of L73.end L130.end
  measures "d120" distance of L74.end L134.end
  measures "d121" distance of L66.end L136.end
  measures "d122" distance of L59.end L138.end
  measures "d123" distance of L57.end L140.end
  measures "d124" distance of L58.end L142.end
  measures "d125" distance of L124.end L154.end
  measures "d126" distance of L118.end L156.end
  measures "d127" distance of L112.end L158.end
  measures "d128" distance of L111.end L160.end
  measures "d129" distance of L117.end L162.end
  measures "d130" distance of L123.end L164.end
extrude "Extrude11" cut sketch "Sketch7" against normal blind 10 contours L124 L127 E6 E11 | L165 E11 L176 L177 | L165 E11 L176 L177 | L165 E11 L176 L177 | L165 E11 L176 L177 | L131 E0 L132 L133 | L74 L77 L88 L94 E0 E1 | L131 E0 L132 L133 | L131 E0 L132 L133 | L131 E0 L132 L133 | L155 E6 L166 L167 | L155 E6 L166 L167 | L155 E6 L166 L167 | L155 E6 L166 L167 | L135 E1 L144 L145 | L135 E1 L144 L145 | L135 E1 L144 L145 | L135 E1 L144 L145 | L118 L121 E7 E10 | L163 E10 L174 L175 | L163 E10 L174 L175 | L163 E10 L174 L175 | L163 E10 L174 L175 | L139 E2 L146 L147 | L139 E2 L146 L147 | L66 L70 L91 L98 E2 E3 | L139 E2 L146 L147 | L157 E7 L168 L169 | L157 E7 L168 L169 | L157 E7 L168 L169 | L157 E7 L168 L169 | L139 E2 L146 L147 | L137 E3 L148 L149 | L137 E3 L148 L149 | L137 E3 L148 L149 | L137 E3 L148 L149 | L159 L170 L171 E9 L173 | L159 L170 L171 E9 L173 | L159 L161 E8 L170 L171 E9 L172 L173 | L159 L161 E8 L170 L171 E9 L172 L173 | L161 E8 L171 L172 L173 | L161 E8 L171 L172 L173 | L141 L143 E4 L150 L151 E5 L152 L153 | L143 L150 L151 E5 L153 | L143 L150 L151 E5 L153 | L141 L143 E4 L150 L151 E5 L152 L153 | L141 E4 L151 L152 L153 | L141 E4 L151 L152 L153